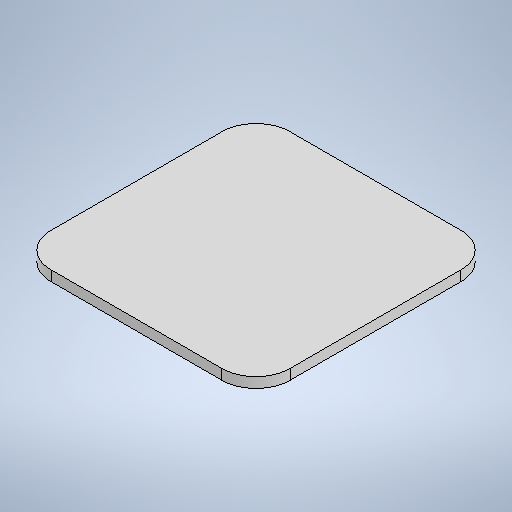
# Autodesk Inventor part: PNS-682 leg plate for filter
Saved by Autodesk Inventor 2025 (Build 290162010, 162A)
## iProperties
Created: 2025-02-20
Part Number: PNS-682 leg plate for filter
Material: Stainless Steel
Document SubType Name: Sheet Metal
Designer: user
Mass: 924.319 g
Surface Area: 416.673 cm^2
Volume: 115.54 cm^3
Density: 8 g/cm^3
Sheet Metal Rule: AISI304 3mm Die 32
Sheet Metal Width: 140,000 mm
Sheet Metal Length: 140,000 mm
Sheet Metal Area: 19600,000 mm^2
Appearance: Default
Flat Pattern Width: 14 cm
Flat Pattern Length: 14 cm
Flat Pattern Area: 196 cm^2
Author: user
Autodesk Inventor part; units mm, degrees
ref_plane "YZ Plane" through (0, 0, 0) normal (1, 0, 0) x (0, 1, 0)
ref_plane "XZ Plane" through (0, 0, 0) normal (0, 1, 0) x (-1, 0, 0)
ref_plane "XY Plane" through (0, 0, 0) normal (0, 0, 1) x (1, 0, 0)
sketch "Sketch1" plane through (0, 0, 0) normal (0, 0, 1) x (1, 0, 0)
  line L0 (-70, -70) -> (70, -70)
  line L1 (70, -70) -> (70, 70)
  line L2 (70, 70) -> (-70, 70)
  line L3 (-70, 70) -> (-70, -70)
  line L4 (-70, -70) -> (70, 70) construction
  line L5 (70, -70) -> (-70, 70) construction
  point P0 (0, 0)
  dimension "d0" = 140
  dimension "d1" = 140
  measures "d0" distance of L2.end L1.end
  measures "d1" distance of L1.end L0.end
extrude "Plate1" add sketch "Sketch1" along normal blind 6
fillet "Corner Round1" radius 20 4 edges at (70, -70, 3) (-70, -70, 3) (-70, 70, 3) (70, 70, 3)
equation "\"d0\" = d1"
equation "\"d2\" = Thickness"
equation "\"BendReliefWidth\" = Thickness"
equation "\"BendReliefDepth\" = 0.5 * Thickness"
equation "\"CornerReliefSize\" = 4 * Thickness"
equation "\"MinimumRemnant\" = 2 * Thickness"
equation "\"TransitionRadius\" = BendRadius"
equation "\"JacobiRadiusSize\" = BendRadius"
equation "\"GapSize\" = Thickness"
equation "\"Thickness\" = 6"
equation "\"BendRadius\" = 5"
body "Solid1"
